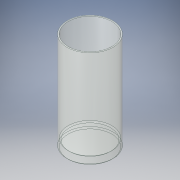
# Autodesk Inventor part: Glas
Saved by Autodesk Inventor 2019 (Build 230136000, 136)
## iProperties
Created: 2018-09-20
Part Number: Glas
Material: Glas
Document SubType Name: Modeling
Designer: nico-
Density: 2.18 g/cm^3
Appearance: Klar
Author: nico-
Autodesk Inventor part; units mm, degrees
ref_plane "YZ Plane" through (0, 0, 0) normal (1, 0, 0) x (0, 1, 0)
ref_plane "XZ Plane" through (0, 0, 0) normal (0, 1, 0) x (-1, 0, 0)
ref_plane "XY Plane" through (0, 0, 0) normal (0, 0, 1) x (1, 0, 0)
sketch "Skizze2" plane through (0, 0, 0) normal (0, 1, 0) x (-1, 0, 0)
  circle A0 centre (0, 0) radius 37.5
  dimension "d0" = 75
  constraints: 1 centre point, 1 coincident
  measures "d0" diameter of A0
extrude "Extrusion1" add sketch "Skizze2" along normal blind 160
sketch "Skizze3" plane through (0, 160, 0) normal (0, 1, 0) x (1, 0, 0)
  circle A0 centre (0, 0) radius 35.5
  dimension "d3" = 71
  constraints: 1 centre point, 1 coincident
  measures "d3" diameter of A0
extrude "Extrusion2" cut sketch "Skizze3" against normal blind 150
fillet "Rundung1" radius 1 2 edges at (37.5, 160, 0) (-35.5, 160, 0)
fillet "Rundung2" radius 2 1 edges at (37.5, 0, 0)
fillet "Rundung3" radius 2 1 edges at (-35.5, 10, 0)
